Autodesk Fusion 360 part; units mm, degrees
note: some values were not read from the file. Set by a fixed rule: which face or edge a step refers to.
(part 2 of 3)
extrude "押し出し2" add sketch "スケッチ2" against normal blind 1 contours A6 L107 L108 A82 | L5 L109 L110 L111 A82 | L5 A6 L108 L109 L110 A82 | L108 A82 A83 L112 | A82 A83 L112 L113 | L110 A82 A83 L113 | L108 L110 A82 A83 | L7 A9 L136 L137 A90 L141 | L7 L136 L137 L138 A90 | A9 A90 L141 L142 | A90 A91 L140 L141 | L136 A90 A91 L141 | L136 A90 A91 L139 | A90 A91 L139 L140 | A11 A80 L100 L103 | A11 L10 L99 A80 L100 L101 | A80 L102 L104 A81 | A80 L100 L102 A81 | L10 L99 A80 L101 L105 | L99 A80 L100 A81 | L99 A80 L104 A81 | L13 A88 L133 L134 L135 | L13 A14 A88 L130 L133 L135 | A88 A89 L131 L132 | A88 A89 L131 L133 | A14 L129 A88 L130 | A88 A89 L130 L132 | A88 A89 L130 L133 | A20 L97 L98 A79 | L15 L94 L97 A79 | L94 L95 L96 L98 A79 | L15 L94 L98 A79 | A20 L92 L93 A78 | L89 L91 L93 A78 | L94 L96 L97 A79 | A21 L97 L98 A79 | L19 L89 L92 A78 | L89 L90 L91 L92 A78 | L19 L89 L93 A78 | A22 L92 L93 A78 | A30 A84 L120 L121 L143 A92 L144 | L22 L115 L116 L117 A84 A92 L147 L148 L149 | L22 A30 L116 L117 A84 L120 A92 L144 L147 L149 | A84 A85 L119 L120 A92 A93 L144 L146 | A84 A85 L118 L119 A92 A93 L145 L146 | L116 A84 A85 L118 A92 A93 L145 L147 | L116 A84 A85 L120 A92 A93 L144 L147 | A33 L72 L73 A74 | L24 L69 L72 A74 | L69 L71 L73 A74 | L24 L69 L73 A74 | A33 L77 L78 A75 | L74 L75 L76 L78 A75 | L69 L70 L72 A74 | A34 L72 L73 A74 | L28 L74 L77 A75 | L74 L76 L77 A75 | L28 L74 L78 A75 | A35 L77 L78 A75 | A46 L122 L123 A86 A94 L155 L156 | A46 L36 L123 A86 L126 L127 L150 L151 A94 L155 | A86 A87 L124 L125 A94 A95 L153 L154 | L123 A86 A87 L125 A94 A95 L154 L155 | L36 A86 L126 L127 L128 L150 L151 L152 A94 | L123 A86 A87 L127 L150 A94 A95 L155 | A86 A87 L124 L127 L150 A94 A95 L153 | L42 A96 L161 L162 L163 | L42 A54 A96 L158 L161 L163 | A96 A97 L159 L160 | A96 A97 L159 L161 | A54 L157 A96 L158 | A96 A97 L158 L160 | A96 A97 L158 L161 | A58 A98 L169 L170 | A58 L47 L164 L165 A98 L169 | A98 A99 L167 L168 | A98 A99 L168 L169 | L47 L164 L165 L166 A98 | L164 A98 A99 L169 | L164 A98 A99 L167 | A61 L82 L83 A76 | L50 L79 L82 A76 | L50 L79 L83 A76 | L79 L80 L81 L83 A76 | A59 L82 L83 A76 | A61 L87 L88 A77 | L84 L86 L87 A77 | L79 L81 L82 A76 | L54 L84 L88 A77 | L84 L85 L86 L88 A77 | L54 L84 L87 A77 | A60 L87 L88 A77
sketch "スケッチ3" plane through (0, 0, 0) normal (0, 0, -1) x (1, 0, 0)
  circle A0 centre (-48.1818, -92.7295) radius 1.65
  circle A1 centre (48.1818, -92.7295) radius 1.65
  circle A2 centre (-55.172, 39.2975) radius 1.65
  circle A3 centre (48.1818, 92.7295) radius 1.65
  circle A4 centre (42.7658, -42.7658) radius 1.45
  arc A5 (35.8727, 82.5418) -> (8, 89.6437) centre (0, 0) ccw
  line L0 (35.8727, 82.5418) -> (31.6784, 78.3474)
  line L1 (31.6784, 78.3474) -> (45.3079, 64.7179)
  line L2 (45.3079, 64.7179) -> (31.945, 51.3551)
  arc A6 (31.945, 51.3551) -> (8, 59.9486) centre (0, 0) ccw
  line L3 (8, 59.9486) -> (8, 89.6437)
  circle A7 centre (-64.0816, 48.207) radius 1.65
  arc A8 (82.5418, -35.8727) -> (89.6437, -8) centre (0, 0) ccw
  line L4 (82.5418, -35.8727) -> (78.3474, -31.6784)
  line L5 (78.3474, -31.6784) -> (64.7179, -45.3079)
  line L6 (64.7179, -45.3079) -> (51.3551, -31.945)
  arc A9 (51.3551, -31.945) -> (59.9486, -8) centre (0, 0) ccw
  line L7 (59.9486, -8) -> (89.6437, -8)
  circle A10 centre (-42.7658, -42.7658) radius 1.45
  circle A11 centre (-48.207, -64.0816) radius 1.65
  circle A12 centre (64.0816, 48.207) radius 1.65
  circle A13 centre (48.207, 64.0816) radius 1.65
  line L8 (61.1824, 48.8434) -> (48.488, 36.149)
  arc A14 (48.488, 36.149) -> (44.8339, 40.5925) centre (0, 0) ccw
  arc A15 (44.8339, 40.5925) -> (40.5925, 44.8339) centre (42.7658, 42.7658) ccw
  arc A16 (40.5925, 44.8339) -> (36.149, 48.488) centre (0, 0) ccw
  line L9 (36.149, 48.488) -> (48.8434, 61.1824)
  line L10 (48.8434, 61.1824) -> (61.1824, 48.8434)
  circle A17 centre (92.7295, -48.1818) radius 1.65
  circle A18 centre (55.172, 39.2975) radius 1.65
  line L11 (31.945, -51.3551) -> (45.3079, -64.7179)
  line L12 (45.3079, -64.7179) -> (37.4856, -72.5402)
  arc A19 (37.4856, -72.5402) -> (10.7877, -59.5101) centre (0, -115.48) ccw
  arc A20 (10.7877, -59.5101) -> (31.945, -51.3551) centre (0, 0) ccw
  circle A21 centre (92.7295, 48.1818) radius 1.65
  circle A22 centre (-39.2975, -55.172) radius 1.65
  arc A23 (-82.5418, 35.8727) -> (-89.6437, 8) centre (0, 0) ccw
  line L13 (-82.5418, 35.8727) -> (-78.3474, 31.6784)
  line L14 (-78.3474, 31.6784) -> (-64.7179, 45.3079)
  line L15 (-64.7179, 45.3079) -> (-51.3551, 31.945)
  arc A24 (-51.3551, 31.945) -> (-59.9486, 8) centre (0, 0) ccw
  line L16 (-59.9486, 8) -> (-89.6437, 8)
  line L17 (-48.488, 36.149) -> (-61.1824, 48.8434)
  line L18 (-61.1824, 48.8434) -> (-48.8434, 61.1824)
  line L19 (-48.8434, 61.1824) -> (-36.149, 48.488)
  arc A25 (-36.149, 48.488) -> (-40.5925, 44.8339) centre (0, 0) ccw
  arc A26 (-40.5925, 44.8339) -> (-44.8339, 40.5925) centre (-42.7658, 42.7658) ccw
  arc A27 (-44.8339, 40.5925) -> (-48.488, 36.149) centre (0, 0) ccw
  circle A28 centre (-42.7658, 42.7658) radius 1.45
  circle A29 centre (55.172, -39.2975) radius 1.65
  circle A30 centre (0, 0) radius 57.48
  circle A31 centre (-48.207, 64.0816) radius 1.65
  circle A32 centre (42.7658, 42.7658) radius 1.45
  circle A33 centre (-55.172, -39.2975) radius 1.65
  circle A34 centre (-64.0816, -48.207) radius 1.65
  line L20 (-33.3352, -82.3475) -> (-38.9921, -76.6906)
  arc A35 (38.9921, -76.6906) -> (-38.9921, -76.6906) centre (0, -115.48) ccw
  line L21 (38.9921, -76.6906) -> (33.3352, -82.3475)
  arc A36 (33.3352, -82.3475) -> (-33.3352, -82.3475) centre (0, -115.48) ccw
  arc A37 (-89.6437, -8) -> (-82.5418, -35.8727) centre (0, 0) ccw
  line L22 (-89.6437, -8) -> (-59.9486, -8)
  arc A38 (-59.9486, -8) -> (-51.3551, -31.945) centre (0, 0) ccw
  line L23 (-51.3551, -31.945) -> (-64.7179, -45.3079)
  line L24 (-64.7179, -45.3079) -> (-78.3474, -31.6784)
  line L25 (-78.3474, -31.6784) -> (-82.5418, -35.8727)
  circle A39 centre (39.2975, 55.172) radius 1.65
  circle A40 centre (-92.7295, -48.1818) radius 1.65
  line L26 (-61.1824, -48.8434) -> (-48.488, -36.149)
  arc A41 (-48.488, -36.149) -> (-44.8339, -40.5925) centre (0, 0) ccw
  arc A42 (-44.8339, -40.5925) -> (-40.5925, -44.8339) centre (-42.7658, -42.7658) ccw
  arc A43 (-40.5925, -44.8339) -> (-36.149, -48.488) centre (0, 0) ccw
  line L27 (-36.149, -48.488) -> (-48.8434, -61.1824)
  line L28 (-48.8434, -61.1824) -> (-61.1824, -48.8434)
  circle A44 centre (48.207, -64.0816) radius 1.65
  circle A45 centre (-48.1818, 92.7295) radius 1.65
  circle A46 centre (39.2975, -55.172) radius 1.65
  arc A47 (89.6437, 8) -> (82.5418, 35.8727) centre (0, 0) ccw
  line L29 (89.6437, 8) -> (59.9486, 8)
  arc A48 (59.9486, 8) -> (51.3551, 31.945) centre (0, 0) ccw
  line L30 (51.3551, 31.945) -> (64.7179, 45.3079)
  line L31 (64.7179, 45.3079) -> (78.3474, 31.6784)
  line L32 (78.3474, 31.6784) -> (82.5418, 35.8727)
  circle A49 centre (-92.7295, 48.1818) radius 1.65
  line L33 (-45.3079, -64.7179) -> (-31.945, -51.3551)
  arc A50 (-31.945, -51.3551) -> (-10.7877, -59.5101) centre (0, 0) ccw
  arc A51 (-10.7877, -59.5101) -> (-37.4856, -72.5402) centre (0, -115.48) ccw
  line L34 (-37.4856, -72.5402) -> (-45.3079, -64.7179)
  circle A52 centre (64.0816, -48.207) radius 1.65
  arc A53 (92.3273, -45.6582) -> (92.3273, 45.6582) centre (0, 0) ccw
  line L35 (92.3273, -45.6582) -> (84.8162, -38.1472)
  arc A54 (84.8162, -38.1472) -> (92.8655, -5) centre (0, 0) ccw
  line L36 (92.8655, -5) -> (60.273, -5)
  line L37 (60.273, -5) -> (60.273, 5)
  line L38 (60.273, 5) -> (92.8655, 5)
  arc A55 (92.8655, 5) -> (84.8162, 38.1472) centre (0, 0) ccw
  line L39 (84.8162, 38.1472) -> (92.3273, 45.6582)
  line L40 (48.488, -36.149) -> (61.1824, -48.8434)
  line L41 (61.1824, -48.8434) -> (48.8434, -61.1824)
  line L42 (48.8434, -61.1824) -> (36.149, -48.488)
  arc A56 (36.149, -48.488) -> (40.5925, -44.8339) centre (0, 0) ccw
  arc A57 (40.5925, -44.8339) -> (44.8339, -40.5925) centre (42.7658, -42.7658) ccw
  arc A58 (44.8339, -40.5925) -> (48.488, -36.149) centre (0, 0) ccw
  arc A59 (-92.3273, 45.6582) -> (-92.3273, -45.6582) centre (0, 0) ccw
  line L43 (-92.3273, 45.6582) -> (-84.8162, 38.1472)
  arc A60 (-84.8162, 38.1472) -> (-92.8655, 5) centre (0, 0) ccw
  line L44 (-92.8655, 5) -> (-60.273, 5)
  line L45 (-60.273, 5) -> (-60.273, -5)
  line L46 (-60.273, -5) -> (-92.8655, -5)
  arc A61 (-92.8655, -5) -> (-84.8162, -38.1472) centre (0, 0) ccw
  line L47 (-84.8162, -38.1472) -> (-92.3273, -45.6582)
  circle A62 centre (-39.2975, 55.172) radius 1.65
  line L48 (-38.1472, 84.8162) -> (-45.6582, 92.3273)
  arc A63 (45.6582, 92.3273) -> (-45.6582, 92.3273) centre (0, 0) ccw
  line L49 (45.6582, 92.3273) -> (38.1472, 84.8162)
  arc A64 (38.1472, 84.8162) -> (5, 92.8655) centre (0, 0) ccw
  line L50 (5, 92.8655) -> (5, 60.273)
  line L51 (5, 60.273) -> (-5, 60.273)
  line L52 (-5, 60.273) -> (-5, 92.8655)
  arc A65 (-5, 92.8655) -> (-38.1472, 84.8162) centre (0, 0) ccw
  line L53 (-31.945, 51.3551) -> (-45.3079, 64.7179)
  line L54 (-45.3079, 64.7179) -> (-31.6784, 78.3474)
  line L55 (-31.6784, 78.3474) -> (-35.8727, 82.5418)
  arc A66 (-8, 89.6437) -> (-35.8727, 82.5418) centre (0, 0) ccw
  line L56 (-8, 89.6437) -> (-8, 59.9486)
  arc A67 (-8, 59.9486) -> (-31.945, 51.3551) centre (0, 0) ccw
  line L57 (-78.3474, -38.7495) -> (-38.7495, -78.3474)
  line L58 (-38.7495, -78.3474) -> (-53.9574, -93.5553)
  arc A68 (-53.9574, -93.5553) -> (-42.0574, -99.4745) centre (0, 0) ccw
  arc A69 (42.0574, -99.4745) -> (-42.0574, -99.4745) centre (0, -115.48) ccw
  arc A70 (42.0574, -99.4745) -> (53.9574, -93.5553) centre (0, 0) ccw
  line L59 (53.9574, -93.5553) -> (38.7495, -78.3474)
  line L60 (38.7495, -78.3474) -> (78.3474, -38.7495)
  line L61 (78.3474, -38.7495) -> (93.5553, -53.9574)
  arc A71 (93.5553, -53.9574) -> (93.5553, 53.9574) centre (0, 0) ccw
  line L62 (93.5553, 53.9574) -> (78.3474, 38.7495)
  line L63 (78.3474, 38.7495) -> (38.7495, 78.3474)
  line L64 (38.7495, 78.3474) -> (53.9574, 93.5553)
  arc A72 (53.9574, 93.5553) -> (-53.9574, 93.5553) centre (0, 0) ccw
  line L65 (-53.9574, 93.5553) -> (-38.7495, 78.3474)
  line L66 (-38.7495, 78.3474) -> (-78.3474, 38.7495)
  line L67 (-78.3474, 38.7495) -> (-93.5553, 53.9574)
  arc A73 (-93.5553, 53.9574) -> (-93.5553, -53.9574) centre (0, 0) ccw
  line L68 (-93.5553, -53.9574) -> (-78.3474, -38.7495)
  line L69 (36.1636, -79.519) -> (37.9314, -81.2868)
  circle A74 centre (37.9314, -81.2868) radius 1.45
  circle A75 centre (37.9314, -81.2868) radius 2.5
  line L70 (37.9314, -81.2868) -> (36.1636, -83.0546)
  line L71 (37.9314, -81.2868) -> (39.6992, -79.519)
  line L72 (39.6992, -79.519) -> (37.9314, -77.7513)
  line L73 (36.1636, -83.0546) -> (34.3959, -81.2868)
  line L74 (-36.1636, -79.519) -> (-37.9314, -81.2868)
  circle A76 centre (-37.9314, -81.2868) radius 2.5
  circle A77 centre (-37.9314, -81.2868) radius 1.45
  line L75 (-37.9314, -81.2868) -> (-39.6992, -79.519)
  line L76 (-37.9314, -81.2868) -> (-36.1636, -83.0546)
  line L77 (-36.1636, -83.0546) -> (-34.3959, -81.2868)
  line L78 (-39.6992, -79.519) -> (-37.9314, -77.7513)
  line L79 (-39.6992, -79.519) -> (-39.8101, -79.4081)
  line L80 (39.6992, -79.519) -> (39.8101, -79.4081)
  circle A78 centre (42.7658, 42.7658) radius 2.55
  line L81 (42.7658, 42.7658) -> (0, 0)
  line L82 (40.9627, 40.9627) -> (39.8079, 39.8079)
  line L83 (40, 40) -> (38.2322, 41.7678)
  line L84 (42.7658, 42.7658) -> (40.9627, 44.5689)
  line L85 (40.9627, 44.5689) -> (38.2322, 41.7678)
  line L86 (42.7658, 42.7658) -> (44.5689, 40.9627)
  line L87 (40, 40) -> (41.8031, 38.1969)
  line L88 (41.8031, 38.1969) -> (44.5689, 40.9627)
  circle A79 centre (-42.7658, 42.7658) radius 2.55
  line L89 (-44.5689, 40.9627) -> (-41.7678, 38.2322)
  line L90 (-40, 40) -> (-41.7678, 38.2322)
  line L91 (-40, 40) -> (-38.1969, 41.8031)
  line L92 (-38.1969, 41.8031) -> (-40.9627, 44.5689)
  line L93 (-42.7658, 42.7658) -> (0, 0)
  circle A80 centre (-42.7658, -42.7658) radius 2.55
  line L94 (-40.9627, -44.5689) -> (-38.2322, -41.7678)
  line L95 (-40, -40) -> (-38.2322, -41.7678)
  line L96 (-40, -40) -> (-41.8031, -38.1969)
  line L97 (-41.8031, -38.1969) -> (-44.5689, -40.9627)
  line L98 (-42.7658, -42.7658) -> (0, 0)
  circle A81 centre (42.7658, -42.7658) radius 2.55
  line L99 (44.5689, -40.9627) -> (41.7678, -38.2322)
  line L100 (40, -40) -> (41.7678, -38.2322)
  line L101 (40, -40) -> (38.1969, -41.8031)
  line L102 (38.1969, -41.8031) -> (40.9627, -44.5689)
  line L103 (42.7658, -42.7658) -> (0, 0)
  dimension "d92" = 2.5
  dimension "d93" = 2.9
  dimension "d94" = 2.5
  dimension "d95" = 2.9
  dimension "d96" = 5.1
  dimension "d97" = 2.5
  dimension "d98" = 2.55
  dimension "d100" = 360
  constraint midpoint L21 L69.start
  constraint perpendicular L21 L69
  constraint coincident L69.end A74.centre
  constraint concentric A74 A75
  constraint coincident L69.start A75
  constraint coincident A75 L70.end
  constraint perpendicular L69 L70
  constraint coincident A75 L71.end
  constraint parallel L70 L71
  constraint coincident L21 L72.end
  constraint tangent A75 L72
  constraint coincident L21 L73.end
  constraint tangent A75 L73
  constraint midpoint L20 L74.start
  constraint perpendicular L57 L74
  constraint coincident L74.end A76.centre
  constraint coincident L74.start A76
  constraint concentric A76 A77
  constraint coincident A76 L75.end
  constraint perpendicular L58 L75
  constraint coincident A76 L76.end
  constraint perpendicular L74 L76
  constraint coincident L20 L77.end
  constraint tangent A76 L77
  constraint coincident L20 L78.end
  constraint tangent A76 L78
  constraint coincident L58 L79.end
  constraint perpendicular L58 L79
  constraint coincident L59 L80.end
  constraint perpendicular L59 L80
  constraint concentric A15 A78
  constraint coincident A15.centre A32.centre
  constraint coincident L81 L82.start
  constraint coincident A78 L82.start
  constraint coincident L81 L82.end
  constraint coincident L82 L83.start
  constraint perpendicular L82 L83
  constraint coincident A78 L84.end
  constraint perpendicular L81 L84
  constraint coincident A78 L86.end
  constraint perpendicular L81 L86
  constraint perpendicular L82 L87
  measures "d92" distance of L69.start L69.end
  measures "d93" diameter of A74
  measures "d94" distance of L74.start L74.end
  measures "d95" diameter of A77
  measures "d96" diameter of A78
  measures "d97" distance of L83.start L83.end
  measures "d98" distance of L83.start L87.end
extrude "押し出し3" cut sketch "スケッチ3" against normal blind 1 contours A30 A78 L81 L82 L88 | A30 A81 L99 L103 | A30 A78 L81 L82 L85 | A32 A78 L84 L86 | A32 A78 L81 L86 | A30 A81 L102 L103 | A32 A78 L81 L84 | A30 A79 L92 L93 | A30 A80 L94 L98 | A30 A79 L89 L93 | A79 | A30 A80 L97 L98 | A80 | L20 A76 L77 | L20 A76 L78 | L74 A76 A77 L76 | L74 A76 A77 L75 | A76 A77 L75 L76 | L21 A75 L73 | L69 A74 A75 L71 | L21 A75 L72 | L69 A74 A75 L70 | A74 A75 L70 L71
extrude "押し出し4" cut 6 faces at (-37.823, 81.023, 0) (-38.2507, 81.8886, 0) (37.8399, 82.0617, 0) (38.2926, 80.9019, 0) (36.7837, 81.6494, 0) (37.3118, 82.3541, 0) along direction (0, 0, 1) blind 2
sketch "スケッチ4" plane through (0, 0, 0) normal (0, 0, -1) x (1, 0, 0)
  line L0 (-78.3474, -38.7495) -> (-38.7495, -78.3474)
  line L1 (-38.7495, -78.3474) -> (-53.9574, -93.5553)
  arc A0 (-53.9574, -93.5553) -> (-42.0574, -99.4745) centre (0, 0) ccw
  arc A1 (42.0574, -99.4745) -> (-42.0574, -99.4745) centre (0, -115.48) ccw
  arc A2 (42.0574, -99.4745) -> (53.9574, -93.5553) centre (0, 0) ccw
  line L2 (53.9574, -93.5553) -> (38.7495, -78.3474)
  line L3 (38.7495, -78.3474) -> (78.3474, -38.7495)
  line L4 (78.3474, -38.7495) -> (93.5553, -53.9574)
  arc A3 (93.5553, -53.9574) -> (93.5553, 53.9574) centre (0, 0) ccw
  line L5 (93.5553, 53.9574) -> (78.3474, 38.7495)
  line L6 (78.3474, 38.7495) -> (38.7495, 78.3474)
  line L7 (38.7495, 78.3474) -> (53.9574, 93.5553)
  arc A4 (53.9574, 93.5553) -> (-53.9574, 93.5553) centre (0, 0) ccw
  line L8 (-53.9574, 93.5553) -> (-38.7495, 78.3474)
  line L9 (-38.7495, 78.3474) -> (-78.3474, 38.7495)
  line L10 (-78.3474, 38.7495) -> (-93.5553, 53.9574)
  arc A5 (-93.5553, 53.9574) -> (-93.5553, -53.9574) centre (0, 0) ccw
  line L11 (-93.5553, -53.9574) -> (-78.3474, -38.7495)
  line L12 (-31.945, 51.3551) -> (-45.3079, 64.7179)
  line L13 (-45.3079, 64.7179) -> (-31.6784, 78.3474)
  line L14 (-31.6784, 78.3474) -> (-35.8727, 82.5418)
  arc A6 (-8, 89.6437) -> (-35.8727, 82.5418) centre (0, 0) ccw
  line L15 (-8, 89.6437) -> (-8, 59.9486)
  arc A7 (-8, 59.9486) -> (-31.945, 51.3551) centre (0, 0) ccw
  line L16 (-38.1472, 84.8162) -> (-45.6582, 92.3273)
  arc A8 (45.6582, 92.3273) -> (-45.6582, 92.3273) centre (0, 0) ccw
  line L17 (45.6582, 92.3273) -> (38.1472, 84.8162)
  arc A9 (38.1472, 84.8162) -> (5, 92.8655) centre (0, 0) ccw
  line L18 (5, 92.8655) -> (5, 60.273)
  line L19 (5, 60.273) -> (-5, 60.273)
  line L20 (-5, 60.273) -> (-5, 92.8655)
  arc A10 (-5, 92.8655) -> (-38.1472, 84.8162) centre (0, 0) ccw
  circle A11 centre (-39.2975, 55.172) radius 1.65
  arc A12 (-92.3273, 45.6582) -> (-92.3273, -45.6582) centre (0, 0) ccw
  line L21 (-92.3273, 45.6582) -> (-84.8162, 38.1472)
  arc A13 (-84.8162, 38.1472) -> (-92.8655, 5) centre (0, 0) ccw
  line L22 (-92.8655, 5) -> (-60.273, 5)
  line L23 (-60.273, 5) -> (-60.273, -5)
  line L24 (-60.273, -5) -> (-92.8655, -5)
  arc A14 (-92.8655, -5) -> (-84.8162, -38.1472) centre (0, 0) ccw
  line L25 (-84.8162, -38.1472) -> (-92.3273, -45.6582)
  line L26 (48.488, -36.149) -> (61.1824, -48.8434)
  line L27 (61.1824, -48.8434) -> (48.8434, -61.1824)
  line L28 (48.8434, -61.1824) -> (36.149, -48.488)
  arc A15 (36.149, -48.488) -> (40.5925, -44.8339) centre (0, 0) ccw
  arc A16 (40.5925, -44.8339) -> (44.8339, -40.5925) centre (42.7658, -42.7658) ccw
  arc A17 (44.8339, -40.5925) -> (48.488, -36.149) centre (0, 0) ccw
  arc A18 (92.3273, -45.6582) -> (92.3273, 45.6582) centre (0, 0) ccw
  line L29 (92.3273, -45.6582) -> (84.8162, -38.1472)
  arc A19 (84.8162, -38.1472) -> (92.8655, -5) centre (0, 0) ccw
  line L30 (92.8655, -5) -> (60.273, -5)
  line L31 (60.273, -5) -> (60.273, 5)
  line L32 (60.273, 5) -> (92.8655, 5)
  arc A20 (92.8655, 5) -> (84.8162, 38.1472) centre (0, 0) ccw
  line L33 (84.8162, 38.1472) -> (92.3273, 45.6582)
  circle A21 centre (64.0816, -48.207) radius 1.65
  line L34 (-45.3079, -64.7179) -> (-31.945, -51.3551)
  arc A22 (-31.945, -51.3551) -> (-10.7877, -59.5101) centre (0, 0) ccw
  arc A23 (-10.7877, -59.5101) -> (-37.4856, -72.5402) centre (0, -115.48) ccw
  line L35 (-37.4856, -72.5402) -> (-45.3079, -64.7179)
  circle A24 centre (-92.7295, 48.1818) radius 1.65
  arc A25 (89.6437, 8) -> (82.5418, 35.8727) centre (0, 0) ccw
  line L36 (89.6437, 8) -> (59.9486, 8)
  arc A26 (59.9486, 8) -> (51.3551, 31.945) centre (0, 0) ccw
  line L37 (51.3551, 31.945) -> (64.7179, 45.3079)
  line L38 (64.7179, 45.3079) -> (78.3474, 31.6784)
  line L39 (78.3474, 31.6784) -> (82.5418, 35.8727)
  circle A27 centre (39.2975, -55.172) radius 1.65
  circle A28 centre (-48.1818, 92.7295) radius 1.65
  circle A29 centre (48.207, -64.0816) radius 1.65
  line L40 (-61.1824, -48.8434) -> (-48.488, -36.149)
  arc A30 (-48.488, -36.149) -> (-44.8339, -40.5925) centre (0, 0) ccw
  arc A31 (-44.8339, -40.5925) -> (-40.5925, -44.8339) centre (-42.7658, -42.7658) ccw
  arc A32 (-40.5925, -44.8339) -> (-36.149, -48.488) centre (0, 0) ccw
  line L41 (-36.149, -48.488) -> (-48.8434, -61.1824)
  line L42 (-48.8434, -61.1824) -> (-61.1824, -48.8434)
  circle A33 centre (-92.7295, -48.1818) radius 1.65
  circle A34 centre (39.2975, 55.172) radius 1.65
  arc A35 (-89.6437, -8) -> (-82.5418, -35.8727) centre (0, 0) ccw
  line L43 (-89.6437, -8) -> (-59.9486, -8)
  arc A36 (-59.9486, -8) -> (-51.3551, -31.945) centre (0, 0) ccw
  line L44 (-51.3551, -31.945) -> (-64.7179, -45.3079)
  line L45 (-64.7179, -45.3079) -> (-78.3474, -31.6784)
  line L46 (-78.3474, -31.6784) -> (-82.5418, -35.8727)
  line L47 (-34.3959, -81.2868) -> (-36.1636, -83.0546)
  arc A37 (-39.6992, -79.519) -> (-36.1636, -83.0546) centre (-37.9314, -81.2868) ccw
  line L48 (-39.6992, -79.519) -> (-37.9314, -77.7513)
  line L49 (-37.9314, -77.7513) -> (-38.9921, -76.6906)
  arc A38 (38.9921, -76.6906) -> (-38.9921, -76.6906) centre (0, -115.48) ccw
  line L50 (38.9921, -76.6906) -> (37.9314, -77.7513)
  line L51 (37.9314, -77.7513) -> (39.6992, -79.519)
  arc A39 (36.1636, -83.0546) -> (39.6992, -79.519) centre (37.9314, -81.2868) ccw
  line L52 (36.1636, -83.0546) -> (34.3959, -81.2868)
  line L53 (34.3959, -81.2868) -> (33.3352, -82.3475)
  arc A40 (33.3352, -82.3475) -> (-33.3352, -82.3475) centre (0, -115.48) ccw
  line L54 (-33.3352, -82.3475) -> (-34.3959, -81.2868)
  circle A41 centre (-64.0816, -48.207) radius 1.65
  circle A42 centre (-55.172, -39.2975) radius 1.65
  circle A43 centre (-48.207, 64.0816) radius 1.65
  circle A44 centre (55.172, -39.2975) radius 1.65
  line L55 (-48.488, 36.149) -> (-61.1824, 48.8434)
  line L56 (-61.1824, 48.8434) -> (-48.8434, 61.1824)
  line L57 (-48.8434, 61.1824) -> (-36.149, 48.488)
  arc A45 (-36.149, 48.488) -> (-40.5925, 44.8339) centre (0, 0) ccw
  arc A46 (-40.5925, 44.8339) -> (-44.8339, 40.5925) centre (-42.7658, 42.7658) ccw
  arc A47 (-44.8339, 40.5925) -> (-48.488, 36.149) centre (0, 0) ccw
  arc A48 (-82.5418, 35.8727) -> (-89.6437, 8) centre (0, 0) ccw
  line L58 (-82.5418, 35.8727) -> (-78.3474, 31.6784)
  line L59 (-78.3474, 31.6784) -> (-64.7179, 45.3079)
  line L60 (-64.7179, 45.3079) -> (-51.3551, 31.945)
  arc A49 (-51.3551, 31.945) -> (-59.9486, 8) centre (0, 0) ccw
  line L61 (-59.9486, 8) -> (-89.6437, 8)
  circle A50 centre (-39.2975, -55.172) radius 1.65
  circle A51 centre (92.7295, 48.1818) radius 1.65
  line L62 (31.945, -51.3551) -> (45.3079, -64.7179)
  line L63 (45.3079, -64.7179) -> (37.4856, -72.5402)
  arc A52 (37.4856, -72.5402) -> (10.7877, -59.5101) centre (0, -115.48) ccw
  arc A53 (10.7877, -59.5101) -> (31.945, -51.3551) centre (0, 0) ccw
  circle A54 centre (55.172, 39.2975) radius 1.65
  circle A55 centre (92.7295, -48.1818) radius 1.65
  line L64 (61.1824, 48.8434) -> (48.488, 36.149)
  arc A56 (48.488, 36.149) -> (44.8339, 40.5925) centre (0, 0) ccw
  arc A57 (44.8339, 40.5925) -> (40.5925, 44.8339) centre (42.7658, 42.7658) ccw
  arc A58 (40.5925, 44.8339) -> (36.149, 48.488) centre (0, 0) ccw
  line L65 (36.149, 48.488) -> (48.8434, 61.1824)
  line L66 (48.8434, 61.1824) -> (61.1824, 48.8434)
  circle A59 centre (48.207, 64.0816) radius 1.65
  circle A60 centre (64.0816, 48.207) radius 1.65
  circle A61 centre (-48.207, -64.0816) radius 1.65
  arc A62 (82.5418, -35.8727) -> (89.6437, -8) centre (0, 0) ccw
  line L67 (82.5418, -35.8727) -> (78.3474, -31.6784)
  line L68 (78.3474, -31.6784) -> (64.7179, -45.3079)
  line L69 (64.7179, -45.3079) -> (51.3551, -31.945)
  arc A63 (51.3551, -31.945) -> (59.9486, -8) centre (0, 0) ccw
  line L70 (59.9486, -8) -> (89.6437, -8)
  circle A64 centre (-64.0816, 48.207) radius 1.65
  arc A65 (35.8727, 82.5418) -> (8, 89.6437) centre (0, 0) ccw
  line L71 (35.8727, 82.5418) -> (31.6784, 78.3474)
  line L72 (31.6784, 78.3474) -> (45.3079, 64.7179)
  line L73 (45.3079, 64.7179) -> (31.945, 51.3551)
  arc A66 (31.945, 51.3551) -> (8, 59.9486) centre (0, 0) ccw
  line L74 (8, 59.9486) -> (8, 89.6437)
  circle A67 centre (48.1818, 92.7295) radius 1.65
  circle A68 centre (-55.172, 39.2975) radius 1.65
  circle A69 centre (48.1818, -92.7295) radius 1.65
  circle A70 centre (-48.1818, -92.7295) radius 1.65
  line L75 (-44.5689, -40.9627) -> (-42.4076, -38.8014)
  arc A71 (-42.3812, 38.8302) -> (-42.4076, -38.8014) centre (0, 0) ccw
  line L76 (-42.3812, 38.8302) -> (-44.5689, 40.9627)
  arc A72 (-40.9627, 44.5689) -> (-44.5689, 40.9627) centre (-42.7658, 42.7658) ccw
  line L77 (-40.9627, 44.5689) -> (-38.8014, 42.4076)
  arc A73 (38.8302, 42.3812) -> (-38.8014, 42.4076) centre (0, 0) ccw
  line L78 (38.8302, 42.3812) -> (40.9627, 44.5689)
  arc A74 (44.5689, 40.9627) -> (40.9627, 44.5689) centre (42.7658, 42.7658) ccw
  line L79 (44.5689, 40.9627) -> (42.4076, 38.8014)
  arc A75 (42.3812, -38.8302) -> (42.4076, 38.8014) centre (0, 0) ccw
  line L80 (42.3812, -38.8302) -> (44.5689, -40.9627)
  arc A76 (40.9627, -44.5689) -> (44.5689, -40.9627) centre (42.7658, -42.7658) ccw
  line L81 (40.9627, -44.5689) -> (38.8014, -42.4076)
  arc A77 (-38.8302, -42.3812) -> (38.8014, -42.4076) centre (0, 0) ccw
  line L82 (-38.8302, -42.3812) -> (-40.9627, -44.5689)
  arc A78 (-44.5689, -40.9627) -> (-40.9627, -44.5689) centre (-42.7658, -42.7658) ccw
  line L83 (0, -60.48) -> (0, -59.48)
  line L84 (0, -59.48) -> (7, -59.48)
  line L85 (7, -59.48) -> (7, -60.9273)
  line L86 (0, -59.48) -> (-7, -59.48)
  line L87 (-7, -59.48) -> (-7, -60.9273)
  dimension "d112" = 1
  dimension "d113" = 7
  dimension "d114" = 7
  constraint midpoint A38 L83.start
  constraint vertical L83
  constraint perpendicular L83 L84
  constraint coincident A38 L85.end
  constraint perpendicular L84 L85
  constraint perpendicular L83 L86
  constraint coincident A38 L87.end
  constraint perpendicular L86 L87
  measures "d112" distance of L83.start L83.end
  measures "d113" distance of L83.end L84.end
  measures "d114" distance of L83.end L86.end
extrude "押し出し5" cut sketch "スケッチ4" against normal blind 2 contours A38 L83 L86 L87 | A38 L83 L84 L85
fillet "フィレット2" radius 3 15 edges at (93.5553, 53.9574, 1) (78.3474, 38.7495, 1) (38.7495, 78.3474, 1) (53.9574, 93.5553, 1) (93.5553, -53.9574, 1) (78.3474, -38.7495, 1) (38.7495, -78.3474, 1) (53.9574, -93.5553, 1) (-53.9574, -93.5553, 1) (-93.5553, -53.9574, 1) (-78.3474, -38.7495, 1) (-93.5553, 53.9574, 1) (-78.3474, 38.7495, 1) (-38.7495, 78.3474, 1) (-53.9574, 93.5553, 1)
fillet "フィレット2" radius 3 2 edges at (-37.4856, 72.5402, 1) (37.4856, 72.5402, 1)
fillet "フィレット2" radius 3 1 edges at (-38.7495, -78.3474, 1)
fillet "フィレット3" radius 3 23 edges at (48.488, -36.149, 1) (61.1824, -48.8434, 1) (64.7179, -45.3079, 1) (48.8434, -61.1824, 1) (45.3079, -64.7179, 1) (36.149, -48.488, 1) (64.7179, 45.3079, 1) (61.1824, 48.8434, 1) (48.488, 36.149, 1) (36.149, 48.488, 1) (48.8434, 61.1824, 1) (45.3079, 64.7179, 1) (-36.149, 48.488, 1) (-48.8434, 61.1824, 1) (-48.488, 36.149, 1) (-61.1824, 48.8434, 1) (-64.7179, 45.3079, 1) (-64.7179, -45.3079, 1) (-61.1824, -48.8434, 1) (-45.3079, -64.7179, 1) (-48.8434, -61.1824, 1) (-36.149, -48.488, 1) (-48.488, -36.149, 1)
fillet "フィレット3" radius 3 1 edges at (-45.3079, 64.7179, 1)
fillet "フィレット5" radius 3 4 edges at (44.8339, 40.5925, 1) (40.5925, 44.8339, 1) (42.3812, 38.8302, 0.5) (38.8014, 42.4076, 0.5)
fillet "フィレット6" radius 3 12 edges at (44.8339, -40.5925, 1) (42.4076, -38.8014, 0.5) (38.8302, -42.3812, 0.5) (40.5925, -44.8339, 1) (-40.5925, -44.8339, 1) (-38.8014, -42.4076, 0.5) (-42.3812, -38.8302, 0.5) (-44.8339, -40.5925, 1) (-40.5925, 44.8339, 1) (-38.8302, 42.3812, 0.5) (-42.4076, 38.8014, 0.5) (-44.8339, 40.5925, 1)
fillet "フィレット7" radius 2 2 edges at (10.7877, 59.5101, 1) (-10.7877, 59.5101, 1)
fillet "フィレット7" radius 5 6 edges at (5, -92.8655, 1) (-5, -92.8655, 1) (92.8655, -5, 1) (92.8655, 5, 1) (-92.8655, -5, 1) (-92.8655, 5, 1)
fillet "フィレット8" radius 2 12 edges at (89.6437, -8, 1) (89.6437, 8, 1) (60.273, 5, 1) (60.273, -5, 1) (-89.6437, -8, 1) (-89.6437, 8, 1) (-60.273, 5, 1) (-60.273, -5, 1) (-5, -60.273, 1) (5, -60.273, 1) (8, -89.6437, 1) (-8, -89.6437, 1)
fillet "フィレット9" radius 2 2 edges at (45.6582, -92.3273, 0.5) (38.1472, -84.8162, 0.5)
fillet "フィレット9" radius 2 10 edges at (-38.1472, -84.8162, 0.5) (-45.6582, -92.3273, 0.5) (92.3273, -45.6582, 0.5) (84.8162, -38.1472, 0.5) (92.3273, 45.6582, 0.5) (84.8162, 38.1472, 0.5) (-84.8162, 38.1472, 0.5) (-92.3273, 45.6582, 0.5) (-84.8162, -38.1472, 0.5) (-92.3273, -45.6582, 0.5)
fillet "フィレット10" radius 8 6 edges at (78.3474, 31.6784, 1) (78.3474, -31.6784, 1) (31.6784, -78.3474, 1) (-31.6784, -78.3474, 1) (-78.3474, -31.6784, 1) (-78.3474, 31.6784, 1)
fillet "フィレット11" radius 2 4 edges at (-33.3352, 82.3475, 1) (-38.9921, 76.6906, 1) (38.9921, 76.6906, 1) (33.3352, 82.3475, 1)
fillet "フィレット12" radius 2 2 edges at (7, 59.48, 1) (-7, 59.48, 1)
fillet "フィレット13" radius 2 2 edges at (7, 60.9273, 1) (-7, 60.9273, 1)
fillet "フィレット13" radius 2 1 edges at (82.5418, -35.8727, 1)
fillet "フィレット15" radius 2 6 edges at (59.9486, 8, 1) (59.9486, -8, 1) (8, -59.9486, 1) (-8, -59.9486, 1) (-59.9486, -8, 1) (-59.9486, 8, 1)
fillet "フィレット15" radius 2 5 edges at (82.5418, 35.8727, 1) (-82.5418, -35.8727, 1) (-82.5418, 35.8727, 1) (-35.8727, -82.5418, 1) (35.8727, -82.5418, 1)
extrude "押し出し6" add 8 faces at (54.1021, 33.4894, 1) (33.4582, 54.0752, 1) (-33.4582, 54.0752, 1) (-54.1021, 33.4894, 1) (-54.1021, -33.4894, 1) (-33.4582, -54.0752, 1) (33.4582, -54.0752, 1) (54.1021, -33.4894, 1) along direction (0, 0, -1) blind 1
fillet "フィレット17" radius 5 8 edges at (55.4793, 36.0692, 1) (36.0692, 55.4793, 1) (-36.0692, 55.4793, 1) (-55.4793, 36.0692, 1) (-55.4793, -36.0692, 1) (-36.0692, -55.4793, 1) (36.0692, -55.4793, 1) (55.4793, -36.0692, 1)
fillet "フィレット18" radius 2 8 edges at (-54.6959, -25.8106, 1) (-25.8106, -54.6959, 1) (25.8106, -54.6959, 1) (54.6959, -25.8106, 1) (54.6959, 25.8106, 1) (25.8106, 54.6959, 1) (-25.8106, 54.6959, 1) (-54.6959, 25.8106, 1)
fillet "フィレット19" radius 2 12 edges at (-94.5642, 40.8241, 1.5) (-86.8909, 33.1508, 1.5) (-86.8909, -33.1508, 1.5) (-94.5642, -40.8241, 1.5) (-40.8241, -94.5642, 1.5) (-33.1508, -86.8909, 1.5) (40.8241, -94.5642, 1.5) (33.1508, -86.8909, 1.5) (86.8909, -33.1508, 1.5) (94.5642, -40.8241, 1.5) (86.8909, 33.1508, 1.5) (94.5642, 40.8241, 1.5)
fillet "フィレット20" radius 1.5 2 edges at (-42.0574, 99.4745, 1) (42.0574, 99.4745, 1)
sketch "スケッチ5" plane through (0, 0, 1) normal (0, 0, -1) x (1, 0, 0)
  arc A0 (85.7845, 39.1155) -> (85.363, 36.9075) centre (87.1987, 37.7012) ccw
  arc A1 (87.3364, 31.9587) -> (85.363, 36.9075) centre (0, 0) ccw
  arc A2 (87.8003, 34.0602) -> (87.3364, 31.9587) centre (89.2146, 32.646) ccw
  line L0 (87.8003, 34.0602) -> (92.4483, 38.7081)
  arc A3 (95.7211, 38.0324) -> (92.4483, 38.7081) centre (93.8625, 37.2939) ccw
  arc A4 (95.7211, 38.0324) -> (93.5579, 43.0803) centre (0, 0) ccw
  arc A5 (93.5579, 43.0803) -> (90.3271, 43.658) centre (91.7413, 42.2438) ccw
  line L1 (90.3271, 43.658) -> (85.7845, 39.1155)
  circle A6 centre (89.6381, 39.4713) radius 1.45
  line L2 (89.6381, 39.4713) -> (87.8893, 41.2202)
  constraint coincident A6.centre L2.start
  constraint coincident L1 L2.end
  constraint perpendicular L1 L2
sketch "スケッチ6" plane through (0, 0, 2) normal (0, 0, 1) x (-1, 0, 0)
  arc A0 (6.6797, -60.2824) -> (7.9909, -61.0636) centre (8.2815, -59.0848) ccw
  arc A1 (37.5046, -75.2506) -> (7.9909, -61.0636) centre (0, -115.48) ccw
  arc A2 (37.555, -78.1277) -> (37.5046, -75.2506) centre (36.1408, -76.7135) ccw
  line L0 (37.555, -78.1277) -> (34.7247, -80.958)
  arc A3 (31.9509, -81.0106) -> (34.7247, -80.958) centre (33.3105, -79.5438) ccw
  arc A4 (31.9509, -81.0106) -> (-31.9509, -81.0106) centre (0, -115.48) ccw
  arc A5 (-34.7247, -80.958) -> (-31.9509, -81.0106) centre (-33.3105, -79.5438) ccw
  line L1 (-34.7247, -80.958) -> (-37.555, -78.1277)
  arc A6 (-37.5046, -75.2506) -> (-37.555, -78.1277) centre (-36.1408, -76.7135) ccw
  arc A7 (-7.9909, -61.0636) -> (-37.5046, -75.2506) centre (0, -115.48) ccw
  arc A8 (-7.9909, -61.0636) -> (-6.6797, -60.2824) centre (-8.2815, -59.0848) ccw
  arc A9 (-5.0779, -59.48) -> (-6.6797, -60.2824) centre (-5.0779, -61.48) ccw
  line L2 (-5.0779, -59.48) -> (5.0779, -59.48)
  arc A10 (6.6797, -60.2824) -> (5.0779, -59.48) centre (5.0779, -61.48) ccw
  arc A11 (80.8919, -35.1534) -> (72.8829, -37.1429) centre (78.5398, -42.7998) ccw
  line L3 (72.8829, -37.1429) -> (66.8393, -43.1865)
  arc A12 (62.5966, -43.1865) -> (66.8393, -43.1865) centre (64.7179, -41.0652) ccw
  line L4 (62.5966, -43.1865) -> (58.9846, -39.5745)
  arc A13 (58.6276, -32.9007) -> (58.9846, -39.5745) centre (62.5201, -36.039) ccw
  arc A14 (58.6276, -32.9007) -> (58.4491, -29.5638) centre (56.6814, -31.3316) ccw
  line L5 (58.4491, -29.5638) -> (55.679, -26.7937)
  arc A15 (55.2656, -24.5671) -> (55.679, -26.7937) centre (57.0932, -25.3795) ccw
  arc A16 (55.2656, -24.5671) -> (59.7003, -9.6799) centre (0, 0) ccw
  arc A17 (61.6746, -8) -> (59.7003, -9.6799) centre (61.6746, -10) ccw
  line L6 (61.6746, -8) -> (87.43, -8)
  arc A18 (89.417, -10.2273) -> (87.43, -8) centre (87.43, -10) ccw
  arc A19 (83.3318, -33.9973) -> (89.417, -10.2273) centre (0, 0) ccw
  arc A20 (80.8919, -35.1534) -> (83.3318, -33.9973) centre (81.48, -33.2418) ccw
  arc A21 (-80.8919, 35.1534) -> (-72.8829, 37.1429) centre (-78.5398, 42.7998) ccw
  line L7 (-72.8829, 37.1429) -> (-66.8393, 43.1865)
  arc A22 (-62.5966, 43.1865) -> (-66.8393, 43.1865) centre (-64.7179, 41.0652) ccw
  line L8 (-62.5966, 43.1865) -> (-58.9846, 39.5745)
  arc A23 (-58.6276, 32.9007) -> (-58.9846, 39.5745) centre (-62.5201, 36.039) ccw
  arc A24 (-58.6276, 32.9007) -> (-58.4491, 29.5638) centre (-56.6814, 31.3316) ccw
  line L9 (-58.4491, 29.5638) -> (-55.679, 26.7937)
  arc A25 (-55.2656, 24.5671) -> (-55.679, 26.7937) centre (-57.0932, 25.3795) ccw
  arc A26 (-55.2656, 24.5671) -> (-59.7003, 9.6799) centre (0, 0) ccw
  arc A27 (-61.6746, 8) -> (-59.7003, 9.6799) centre (-61.6746, 10) ccw
  line L10 (-61.6746, 8) -> (-87.43, 8)
  arc A28 (-89.417, 10.2273) -> (-87.43, 8) centre (-87.43, 10) ccw
  arc A29 (-83.3318, 33.9973) -> (-89.417, 10.2273) centre (0, 0) ccw
  arc A30 (-80.8919, 35.1534) -> (-83.3318, 33.9973) centre (-81.48, 33.2418) ccw
  arc A31 (-87.43, -5) -> (-92.3976, -10.5682) centre (-87.43, -10) ccw
  arc A32 (-92.3976, -10.5682) -> (-87.3364, -31.9587) centre (0, 0) ccw
  arc A33 (-87.8003, -34.0602) -> (-87.3364, -31.9587) centre (-89.2146, -32.646) ccw
  line L11 (-87.8003, -34.0602) -> (-92.4483, -38.7081)
  arc A34 (-95.7211, -38.0324) -> (-92.4483, -38.7081) centre (-93.8625, -37.2939) ccw
  arc A35 (-95.7211, 38.0324) -> (-95.7211, -38.0324) centre (0, 0) ccw
  arc A36 (-92.4483, 38.7081) -> (-95.7211, 38.0324) centre (-93.8625, 37.2939) ccw
  line L12 (-92.4483, 38.7081) -> (-87.8003, 34.0602)
  arc A37 (-87.3364, 31.9587) -> (-87.8003, 34.0602) centre (-89.2146, 32.646) ccw
  arc A38 (-87.3364, 31.9587) -> (-92.3976, 10.5682) centre (0, 0) ccw
  arc A39 (-92.3976, 10.5682) -> (-87.43, 5) centre (-87.43, 10) ccw
  line L13 (-87.43, 5) -> (-62.273, 5)
  arc A40 (-60.273, 3) -> (-62.273, 5) centre (-62.273, 3) ccw
  line L14 (-60.273, 3) -> (-60.273, -3)
  arc A41 (-62.273, -5) -> (-60.273, -3) centre (-62.273, -3) ccw
  line L15 (-62.273, -5) -> (-87.43, -5)
  arc A42 (-43.4817, -98.8602) -> (-41.4947, -98.0676) centre (-42.8778, -97.4871) ccw
  arc A43 (41.4947, -98.0676) -> (-41.4947, -98.0676) centre (0, -115.48) ccw
  arc A44 (41.4947, -98.0676) -> (43.4817, -98.8602) centre (42.8778, -97.4871) ccw
  arc A45 (43.4817, -98.8602) -> (50.4167, -95.51) centre (0, 0) ccw
  arc A46 (50.4167, -95.51) -> (51.1376, -90.7356) centre (49.0163, -92.8569) ccw
  line L16 (51.1376, -90.7356) -> (40.8708, -80.4688)
  arc A47 (40.8708, -76.2261) -> (40.8708, -80.4688) centre (42.9921, -78.3474) ccw
  line L17 (40.8708, -76.2261) -> (76.2261, -40.8708)
  arc A48 (80.4688, -40.8708) -> (76.2261, -40.8708) centre (78.3474, -42.9921) ccw
  line L18 (80.4688, -40.8708) -> (90.7356, -51.1376)
  arc A49 (90.7356, -51.1376) -> (95.51, -50.4167) centre (92.8569, -49.0163) ccw
  arc A50 (95.51, -50.4167) -> (95.51, 50.4167) centre (0, 0) ccw
  arc A51 (95.51, 50.4167) -> (90.7356, 51.1376) centre (92.8569, 49.0163) ccw
  line L19 (90.7356, 51.1376) -> (80.4688, 40.8708)
  arc A52 (76.2261, 40.8708) -> (80.4688, 40.8708) centre (78.3474, 42.9921) ccw
  line L20 (76.2261, 40.8708) -> (40.8708, 76.2261)
  arc A53 (40.8708, 80.4688) -> (40.8708, 76.2261) centre (42.9921, 78.3474) ccw
  line L21 (40.8708, 80.4688) -> (51.1376, 90.7356)
  arc A54 (51.1376, 90.7356) -> (50.4167, 95.51) centre (49.0163, 92.8569) ccw
  arc A55 (50.4167, 95.51) -> (-50.4167, 95.51) centre (0, 0) ccw
  arc A56 (-50.4167, 95.51) -> (-51.1376, 90.7356) centre (-49.0163, 92.8569) ccw
  line L22 (-51.1376, 90.7356) -> (-40.8708, 80.4688)
  arc A57 (-40.8708, 76.2261) -> (-40.8708, 80.4688) centre (-42.9921, 78.3474) ccw
  line L23 (-40.8708, 76.2261) -> (-76.2261, 40.8708)
  arc A58 (-80.4688, 40.8708) -> (-76.2261, 40.8708) centre (-78.3474, 42.9921) ccw
  line L24 (-80.4688, 40.8708) -> (-90.7356, 51.1376)
  arc A59 (-90.7356, 51.1376) -> (-95.51, 50.4167) centre (-92.8569, 49.0163) ccw
  arc A60 (-95.51, 50.4167) -> (-95.51, -50.4167) centre (0, 0) ccw
  arc A61 (-95.51, -50.4167) -> (-90.7356, -51.1376) centre (-92.8569, -49.0163) ccw
  line L25 (-90.7356, -51.1376) -> (-80.4688, -40.8708)
  arc A62 (-76.2261, -40.8708) -> (-80.4688, -40.8708) centre (-78.3474, -42.9921) ccw
  line L26 (-76.2261, -40.8708) -> (-40.8708, -76.2261)
  arc A63 (-40.8708, -80.4688) -> (-40.8708, -76.2261) centre (-42.9921, -78.3474) ccw
  line L27 (-40.8708, -80.4688) -> (-51.1376, -90.7356)
  arc A64 (-51.1376, -90.7356) -> (-50.4167, -95.51) centre (-49.0163, -92.8569) ccw
  arc A65 (-50.4167, -95.51) -> (-43.4817, -98.8602) centre (0, 0) ccw
  circle A66 centre (37.9314, -81.2868) radius 1.45
  circle A67 centre (-37.9314, -81.2868) radius 1.45
  circle A68 centre (-31.3316, -56.6814) radius 1.65
  circle A69 centre (56.6814, -31.3316) radius 1.65
  circle A70 centre (-39.4713, 89.6381) radius 1.45
  circle A71 centre (89.6381, -39.4713) radius 1.45
  circle A72 centre (-89.6381, -39.4713) radius 1.45
  circle A73 centre (-56.6814, -31.3316) radius 1.65
  circle A74 centre (-31.3316, 56.6814) radius 1.65
  circle A75 centre (31.3316, -56.6814) radius 1.65
  circle A76 centre (56.6814, 31.3316) radius 1.65
  circle A77 centre (39.4713, 89.6381) radius 1.45
  circle A78 centre (89.6381, 39.4713) radius 1.45
  circle A79 centre (-89.6381, 39.4713) radius 1.45
  circle A80 centre (-56.6814, 31.3316) radius 1.65
  circle A81 centre (31.3316, 56.6814) radius 1.65
  circle A82 centre (-48.1818, -92.7295) radius 1.65
  circle A83 centre (55.172, 39.2975) radius 1.65
  circle A84 centre (-42.7658, 42.7658) radius 1.45
  circle A85 centre (42.7658, 42.7658) radius 1.45
  circle A86 centre (-55.172, 39.2975) radius 1.65
  circle A87 centre (48.1818, 92.7295) radius 1.65
  line L28 (-43.1865, -62.5966) -> (-39.5745, -58.9846)
  arc A88 (-32.9007, -58.6276) -> (-39.5745, -58.9846) centre (-36.039, -62.5201) ccw
  arc A89 (-32.9007, -58.6276) -> (-29.5638, -58.4491) centre (-31.3316, -56.6814) ccw
  line L29 (-29.5638, -58.4491) -> (-26.7937, -55.679)
  arc A90 (-24.5671, -55.2656) -> (-26.7937, -55.679) centre (-25.3795, -57.0932) ccw
  arc A91 (-24.5671, -55.2656) -> (-18.2413, -57.6635) centre (0, 0) ccw
  arc A92 (-18.2058, -61.4656) -> (-18.2413, -57.6635) centre (-18.8446, -59.5704) ccw
  arc A93 (-18.2058, -61.4656) -> (-35.435, -70.833) centre (0, -115.48) ccw
  arc A94 (-39.4214, -70.6044) -> (-35.435, -70.833) centre (-37.3, -68.4831) ccw
  line L30 (-39.4214, -70.6044) -> (-43.1865, -66.8393)
  arc A95 (-43.1865, -62.5966) -> (-43.1865, -66.8393) centre (-41.0652, -64.7179) ccw
  line L31 (50.8737, -38.5347) -> (59.0611, -46.7221)
  arc A96 (59.0611, -50.9647) -> (59.0611, -46.7221) centre (56.9398, -48.8434) ccw
  line L32 (59.0611, -50.9647) -> (50.9647, -59.0611)
  arc A97 (46.7221, -59.0611) -> (50.9647, -59.0611) centre (48.8434, -56.9398) ccw
  line L33 (46.7221, -59.0611) -> (38.5347, -50.8737)
  arc A98 (38.7347, -46.4484) -> (38.5347, -50.8737) centre (40.656, -48.7524) ccw
  arc A99 (38.7347, -46.4484) -> (39.0322, -46.1987) centre (0, 0) ccw
  arc A100 (41.8671, -45.628) -> (39.0322, -46.1987) centre (40.9684, -48.4903) ccw
  arc A101 (41.8671, -45.628) -> (45.628, -41.8671) centre (42.7658, -42.7658) ccw
  arc A102 (46.1987, -39.0322) -> (45.628, -41.8671) centre (48.4903, -40.9684) ccw
  arc A103 (46.1987, -39.0322) -> (46.4484, -38.7347) centre (0, 0) ccw
  arc A104 (50.8737, -38.5347) -> (46.4484, -38.7347) centre (48.7524, -40.656) ccw
  circle A105 centre (39.2975, 55.172) radius 1.65
  circle A106 centre (92.7295, -48.1818) radius 1.65
  line L34 (59.0611, 46.7221) -> (50.8737, 38.5347)
  arc A107 (46.4484, 38.7347) -> (50.8737, 38.5347) centre (48.7524, 40.656) ccw
  arc A108 (46.4484, 38.7347) -> (46.1987, 39.0322) centre (0, 0) ccw
  arc A109 (45.628, 41.8671) -> (46.1987, 39.0322) centre (48.4903, 40.9684) ccw
  arc A110 (45.628, 41.8671) -> (41.8671, 45.628) centre (42.7658, 42.7658) ccw
  arc A111 (39.0322, 46.1987) -> (41.8671, 45.628) centre (40.9684, 48.4903) ccw
  arc A112 (39.0322, 46.1987) -> (38.7347, 46.4484) centre (0, 0) ccw
  arc A113 (38.5347, 50.8737) -> (38.7347, 46.4484) centre (40.656, 48.7524) ccw
  line L35 (38.5347, 50.8737) -> (46.7221, 59.0611)
  arc A114 (50.9647, 59.0611) -> (46.7221, 59.0611) centre (48.8434, 56.9398) ccw
  line L36 (50.9647, 59.0611) -> (59.0611, 50.9647)
  arc A115 (59.0611, 46.7221) -> (59.0611, 50.9647) centre (56.9398, 48.8434) ccw
  circle A116 centre (-48.1818, 92.7295) radius 1.65
  circle A117 centre (64.0816, 48.207) radius 1.65
  circle A118 centre (48.1818, -92.7295) radius 1.65
  arc A119 (-89.417, -10.2273) -> (-83.3318, -33.9973) centre (0, 0) ccw
  arc A120 (-87.43, -8) -> (-89.417, -10.2273) centre (-87.43, -10) ccw
  line L37 (-87.43, -8) -> (-61.6746, -8)
  arc A121 (-59.7003, -9.6799) -> (-61.6746, -8) centre (-61.6746, -10) ccw
  arc A122 (-59.7003, -9.6799) -> (-55.2656, -24.5671) centre (0, 0) ccw
  arc A123 (-55.679, -26.7937) -> (-55.2656, -24.5671) centre (-57.0932, -25.3795) ccw
  line L38 (-55.679, -26.7937) -> (-58.4491, -29.5638)
  arc A124 (-58.4491, -29.5638) -> (-58.6276, -32.9007) centre (-56.6814, -31.3316) ccw
  arc A125 (-58.9846, -39.5745) -> (-58.6276, -32.9007) centre (-62.5201, -36.039) ccw
  line L39 (-58.9846, -39.5745) -> (-62.5966, -43.1865)
  arc A126 (-66.8393, -43.1865) -> (-62.5966, -43.1865) centre (-64.7179, -41.0652) ccw
  line L40 (-66.8393, -43.1865) -> (-72.8829, -37.1429)
  arc A127 (-72.8829, -37.1429) -> (-80.8919, -35.1534) centre (-78.5398, -42.7998) ccw
  arc A128 (-83.3318, -33.9973) -> (-80.8919, -35.1534) centre (-81.48, -33.2418) ccw
  circle A129 centre (-64.0816, 48.207) radius 1.65
  circle A130 centre (-39.2975, 55.172) radius 1.65
  circle A131 centre (64.0816, -48.207) radius 1.65
  circle A132 centre (48.207, 64.0816) radius 1.65
  arc A133 (89.417, 10.2273) -> (83.3318, 33.9973) centre (0, 0) ccw
  arc A134 (87.43, 8) -> (89.417, 10.2273) centre (87.43, 10) ccw
  line L41 (87.43, 8) -> (61.6746, 8)
  arc A135 (59.7003, 9.6799) -> (61.6746, 8) centre (61.6746, 10) ccw
  arc A136 (59.7003, 9.6799) -> (55.2656, 24.5671) centre (0, 0) ccw
  arc A137 (55.679, 26.7937) -> (55.2656, 24.5671) centre (57.0932, 25.3795) ccw
  line L42 (55.679, 26.7937) -> (58.4491, 29.5638)
  arc A138 (58.4491, 29.5638) -> (58.6276, 32.9007) centre (56.6814, 31.3316) ccw
  arc A139 (58.9846, 39.5745) -> (58.6276, 32.9007) centre (62.5201, 36.039) ccw
  line L43 (58.9846, 39.5745) -> (62.5966, 43.1865)
  arc A140 (66.8393, 43.1865) -> (62.5966, 43.1865) centre (64.7179, 41.0652) ccw
  line L44 (66.8393, 43.1865) -> (72.8829, 37.1429)
  arc A141 (72.8829, 37.1429) -> (80.8919, 35.1534) centre (78.5398, 42.7998) ccw
  arc A142 (83.3318, 33.9973) -> (80.8919, 35.1534) centre (81.48, 33.2418) ccw
  line L45 (-59.0611, -46.7221) -> (-50.8737, -38.5347)
  arc A143 (-46.4484, -38.7347) -> (-50.8737, -38.5347) centre (-48.7524, -40.656) ccw
  arc A144 (-46.4484, -38.7347) -> (-46.1987, -39.0322) centre (0, 0) ccw
  arc A145 (-45.628, -41.8671) -> (-46.1987, -39.0322) centre (-48.4903, -40.9684) ccw
  arc A146 (-45.628, -41.8671) -> (-41.8671, -45.628) centre (-42.7658, -42.7658) ccw
  arc A147 (-39.0322, -46.1987) -> (-41.8671, -45.628) centre (-40.9684, -48.4903) ccw
  arc A148 (-39.0322, -46.1987) -> (-38.7347, -46.4484) centre (0, 0) ccw
  arc A149 (-38.5347, -50.8737) -> (-38.7347, -46.4484) centre (-40.656, -48.7524) ccw
  line L46 (-38.5347, -50.8737) -> (-46.7221, -59.0611)
  arc A150 (-50.9647, -59.0611) -> (-46.7221, -59.0611) centre (-48.8434, -56.9398) ccw
  line L47 (-50.9647, -59.0611) -> (-59.0611, -50.9647)
  arc A151 (-59.0611, -46.7221) -> (-59.0611, -50.9647) centre (-56.9398, -48.8434) ccw
  circle A152 centre (-55.172, -39.2975) radius 1.65
  circle A153 centre (-39.2975, -55.172) radius 1.65
  circle A154 centre (-42.7658, -42.7658) radius 1.45
  circle A155 centre (92.7295, 48.1818) radius 1.65
  circle A156 centre (48.207, -64.0816) radius 1.65
  circle A157 centre (-64.0816, -48.207) radius 1.65
  circle A158 centre (39.2975, -55.172) radius 1.65
  line L48 (-50.8737, 38.5347) -> (-59.0611, 46.7221)
  arc A159 (-59.0611, 50.9647) -> (-59.0611, 46.7221) centre (-56.9398, 48.8434) ccw
  line L49 (-59.0611, 50.9647) -> (-50.9647, 59.0611)
  arc A160 (-46.7221, 59.0611) -> (-50.9647, 59.0611) centre (-48.8434, 56.9398) ccw
  line L50 (-46.7221, 59.0611) -> (-38.5347, 50.8737)
  arc A161 (-38.7347, 46.4484) -> (-38.5347, 50.8737) centre (-40.656, 48.7524) ccw
  arc A162 (-38.7347, 46.4484) -> (-39.0322, 46.1987) centre (0, 0) ccw
  arc A163 (-41.8671, 45.628) -> (-39.0322, 46.1987) centre (-40.9684, 48.4903) ccw
  arc A164 (-41.8671, 45.628) -> (-45.628, 41.8671) centre (-42.7658, 42.7658) ccw
  arc A165 (-46.1987, 39.0322) -> (-45.628, 41.8671) centre (-48.4903, 40.9684) ccw
  arc A166 (-46.1987, 39.0322) -> (-46.4484, 38.7347) centre (0, 0) ccw
  arc A167 (-50.8737, 38.5347) -> (-46.4484, 38.7347) centre (-48.7524, 40.656) ccw
  circle A168 centre (-48.207, -64.0816) radius 1.65
  arc A169 (-10.2273, 89.417) -> (-33.9973, 83.3318) centre (0, 0) ccw
  arc A170 (-8, 87.43) -> (-10.2273, 89.417) centre (-10, 87.43) ccw
  line L51 (-8, 87.43) -> (-8, 61.6746)
  arc A171 (-9.6799, 59.7003) -> (-8, 61.6746) centre (-10, 61.6746) ccw
  arc A172 (-9.6799, 59.7003) -> (-24.5671, 55.2656) centre (0, 0) ccw
  arc A173 (-26.7937, 55.679) -> (-24.5671, 55.2656) centre (-25.3795, 57.0932) ccw
  line L52 (-26.7937, 55.679) -> (-29.5638, 58.4491)
  arc A174 (-29.5638, 58.4491) -> (-32.9007, 58.6276) centre (-31.3316, 56.6814) ccw
  arc A175 (-39.5745, 58.9846) -> (-32.9007, 58.6276) centre (-36.039, 62.5201) ccw
  line L53 (-39.5745, 58.9846) -> (-43.1865, 62.5966)
  arc A176 (-43.1865, 66.8393) -> (-43.1865, 62.5966) centre (-41.0652, 64.7179) ccw
  line L54 (-43.1865, 66.8393) -> (-37.1429, 72.8829)
  arc A177 (-37.1429, 72.8829) -> (-35.1534, 80.8919) centre (-42.7998, 78.5398) ccw
  arc A178 (-33.9973, 83.3318) -> (-35.1534, 80.8919) centre (-33.2418, 81.48) ccw
  circle A179 centre (-48.207, 64.0816) radius 1.65
  circle A180 centre (55.172, -39.2975) radius 1.65
  circle A181 centre (0, 0) radius 57.48
  circle A182 centre (42.7658, -42.7658) radius 1.45
  circle A183 centre (-92.7295, -48.1818) radius 1.65
  circle A184 centre (-92.7295, 48.1818) radius 1.65
  line L55 (39.5745, -58.9846) -> (43.1865, -62.5966)
  arc A185 (43.1865, -66.8393) -> (43.1865, -62.5966) centre (41.0652, -64.7179) ccw
  line L56 (43.1865, -66.8393) -> (39.4214, -70.6044)
  arc A186 (35.435, -70.833) -> (39.4214, -70.6044) centre (37.3, -68.4831) ccw
  arc A187 (35.435, -70.833) -> (18.2058, -61.4656) centre (0, -115.48) ccw
  arc A188 (18.2413, -57.6635) -> (18.2058, -61.4656) centre (18.8446, -59.5704) ccw
  arc A189 (18.2413, -57.6635) -> (24.5671, -55.2656) centre (0, 0) ccw
  arc A190 (26.7937, -55.679) -> (24.5671, -55.2656) centre (25.3795, -57.0932) ccw
  line L57 (26.7937, -55.679) -> (29.5638, -58.4491)
  arc A191 (29.5638, -58.4491) -> (32.9007, -58.6276) centre (31.3316, -56.6814) ccw
  arc A192 (39.5745, -58.9846) -> (32.9007, -58.6276) centre (36.039, -62.5201) ccw
  arc A193 (10.5682, 92.3976) -> (5, 87.43) centre (10, 87.43) ccw
  line L58 (5, 87.43) -> (5, 62.273)
  arc A194 (3, 60.273) -> (5, 62.273) centre (3, 62.273) ccw
  line L59 (3, 60.273) -> (-3, 60.273)
  arc A195 (-5, 62.273) -> (-3, 60.273) centre (-3, 62.273) ccw
  line L60 (-5, 62.273) -> (-5, 87.43)
  arc A196 (-5, 87.43) -> (-10.5682, 92.3976) centre (-10, 87.43) ccw
  arc A197 (-10.5682, 92.3976) -> (-31.9587, 87.3364) centre (0, 0) ccw
  arc A198 (-34.0602, 87.8003) -> (-31.9587, 87.3364) centre (-32.646, 89.2146) ccw
  line L61 (-34.0602, 87.8003) -> (-38.7081, 92.4483)
  arc A199 (-38.0324, 95.7211) -> (-38.7081, 92.4483) centre (-37.2939, 93.8625) ccw
  arc A200 (38.0324, 95.7211) -> (-38.0324, 95.7211) centre (0, 0) ccw
  arc A201 (38.7081, 92.4483) -> (38.0324, 95.7211) centre (37.2939, 93.8625) ccw
  line L62 (38.7081, 92.4483) -> (34.0602, 87.8003)
  arc A202 (31.9587, 87.3364) -> (34.0602, 87.8003) centre (32.646, 89.2146) ccw
  arc A203 (31.9587, 87.3364) -> (10.5682, 92.3976) centre (0, 0) ccw
  arc A204 (92.3976, -10.5682) -> (87.43, -5) centre (87.43, -10) ccw
  line L63 (87.43, -5) -> (62.273, -5)
  arc A205 (60.273, -3) -> (62.273, -5) centre (62.273, -3) ccw
  line L64 (60.273, -3) -> (60.273, 3)
  arc A206 (62.273, 5) -> (60.273, 3) centre (62.273, 3) ccw
  line L65 (62.273, 5) -> (87.43, 5)
  arc A207 (87.43, 5) -> (92.3976, 10.5682) centre (87.43, 10) ccw
  arc A208 (92.3976, 10.5682) -> (87.3364, 31.9587) centre (0, 0) ccw
  arc A209 (87.8003, 34.0602) -> (87.3364, 31.9587) centre (89.2146, 32.646) ccw
  line L66 (87.8003, 34.0602) -> (92.4483, 38.7081)
  arc A210 (95.7211, 38.0324) -> (92.4483, 38.7081) centre (93.8625, 37.2939) ccw
  arc A211 (95.7211, -38.0324) -> (95.7211, 38.0324) centre (0, 0) ccw
  arc A212 (92.4483, -38.7081) -> (95.7211, -38.0324) centre (93.8625, -37.2939) ccw
  line L67 (92.4483, -38.7081) -> (87.8003, -34.0602)
  arc A213 (87.3364, -31.9587) -> (87.8003, -34.0602) centre (89.2146, -32.646) ccw